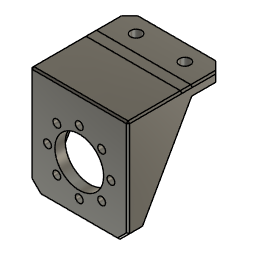
Simple Motor Bracket (Autodesk Fusion 360 design; units mm, degrees)
Autodesk Fusion 360 part; units mm, degrees
sketch "Sketch1" plane through (0, 0, 0) normal (0, 1, 0) x (1, 0, 0)
  circle A0 centre (0, 0) radius 7.5
  circle A1 centre (9.75, 0) radius 1.2
  line L0 (15, -14.8) -> (-15, -14.8)
  line L1 (-15, -14.8) -> (-15, 14.8)
  line L2 (-15, 14.8) -> (15, 14.8)
  line L3 (15, 14.8) -> (15, -14.8)
  line L4 (15, -14.8) -> (-15, 14.8) construction
  line L5 (-15, -14.8) -> (15, 14.8) construction
  line L6 (-15, -14.8) -> (-15, -18)
  line L7 (-15, -18) -> (15, -18)
  line L8 (15, -18) -> (15, -14.8)
  line L9 (12.8, 14.8) -> (12.8, -14.8)
  line L10 (0, 0) -> (0, -2.4)
  circle A2 centre (0, 0) radius 12.5
  circle A3 centre (0, 0) radius 9.75
  line L11 (0, 0) -> (9.75, 0)
  line L12 (1.75, 0) -> (22.5, 0)
  circle A4 centre (6.8943, -6.8943) radius 1.2
  line L13 (0, 0) -> (6.8943, -6.8943)
  line L14 (0, -1.75) -> (0, -22.5)
  circle A5 centre (-6.8943, -6.8943) radius 1.2
  circle A6 centre (-9.75, 0) radius 1.2
  circle A7 centre (0, -9.75) radius 1.2
  circle A8 centre (-6.8943, 6.8943) radius 1.2
  circle A9 centre (0, 9.75) radius 1.2
  circle A10 centre (6.8943, 6.8943) radius 1.2
  line L15 (-12.8, 14.8) -> (-12.8, -14.8)
  dimension "d1" = 15
  dimension "d3" = 2.4
  dimension "d6" = 30
  dimension "d7" = 29.6
  dimension "d8" = 3.2
  dimension "d30" = 2.2
  dimension "d38" = 25
  dimension "d39" = 19.5
  dimension "d40" = 45
  constraint coincident A0.centre L10.start
  constraint horizontal L0
  constraint perpendicular L0 L1
  constraint parallel L0 L2
  constraint parallel L1 L3
  constraint coincident L4 A0.centre
  constraint coincident L5 A0.centre
  constraint perpendicular L1 L7
  constraint perpendicular L6 L7
  constraint perpendicular L7 L8
  constraint coincident L2 L9.start
  constraint coincident L0 L9.end
  constraint perpendicular L0 L9
  constraint concentric A0 A3
  constraint coincident A1.centre A3
  constraint coincident A1.centre L11.end
  constraint parallel L11 L12
  constraint coincident A3 A4.centre
  constraint equal A1 A4
  constraint coincident A4.centre L13.end
  constraint symmetric A1 L14 A6
  constraint symmetric A4 L14 A5
  constraint coincident A3 A7.centre
  constraint coincident L14 A7.centre
  constraint equal A4 A7
  constraint symmetric L11 A4 A10
  constraint symmetric L11 A5 A8
  constraint symmetric L11 A7 A9
  constraint symmetric L9.start L10 L15.start
  constraint symmetric L9.end L10 L15.end
  constraint coincident L10.end L14
  measures "d1" diameter of A0
  measures "d3" diameter of A1
  measures "d6" distance of L1 L3
  measures "d7" distance of L0.start L2.end
  measures "d8" distance of L0 L7
  measures "d30" distance of L3 L9
  measures "d38" diameter of A2
  measures "d39" diameter of A3
  measures "d40" angle of L11 L13
extrude "Extrude1" add sketch "Sketch1" against normal blind 3.2 contours A0 A1 A3 L11 L12 A4 L13 | A0 A1 A3 L11 L12 L14 A5 A6 A7 A8 A9 A10 | A0 A3 A4 L13 L14 A7 | A1 A2 A3 L12 L14 A5 A6 A7 A8 A9 A10 | A1 A2 A3 L12 A4 L14 A7 | L0 L9 A2 L12 L14 | L0 L2 L9 A2 L12 L14 L15 | L0 L3 L9 L12 | L2 L3 L9 L12 | L0 L6 L7 L14 | L0 L7 L8 L14 | L0 L1 L2 L15
extrude "Extrude2" add sketch "Sketch1" along normal blind 26.8 contours L0 L6 L7 L14 | L0 L7 L8 L14
sketch "Sketch2" plane through (0, 0, 18) normal (0, 0, 1) x (-1, 0, 0)
  line L0 (15, -26.8) -> (15, 3.2)
  line L1 (15, 3.2) -> (-15, 3.2)
  line L2 (-15, 3.2) -> (-15, -26.8)
  line L3 (-15, -26.8) -> (15, -26.8)
  dimension "d29" = 0.5
sketch "Sketch3" plane through (0, 0, 18) normal (0, 0, 1) x (-1, 0, 0)
  circle A0 centre (7.5, -21.8) radius 1.7
  line L0 (15, 3.2) -> (-15, 3.2)
  line L1 (0, 0) -> (0, -4)
  circle A1 centre (-7.5, -21.8) radius 1.7
  line L2 (15, -13.4) -> (-15, -13.4)
  line L3 (-15, -13.4) -> (-15, -16.6)
  line L4 (-15, -16.6) -> (15, -16.6)
  line L5 (15, -16.6) -> (15, -13.4)
  line L6 (-15, -26.8) -> (15, -26.8)
  point P0 (-15, 3.2)
  dimension "d13" = 3.4
  dimension "d14" = 25
  dimension "d15" = 7.5
  dimension "d16" = 3.2
  dimension "d17" = 10.2
  constraint coincident L1.start origin
  constraint vertical L1
  constraint symmetric A0 L1 A1
  constraint horizontal L2
  constraint vertical L3
  constraint horizontal L4
  constraint vertical L5
  constraint collinear L0.start L2.start L4.end
  constraint collinear L2.end L3.end P0
  measures "d13" diameter of A0
  measures "d14" distance of A0.centre L0
  measures "d15" distance of A0.centre L1
  measures "d16" distance of L2 L4
  measures "d17" distance of L4 L6
extrude "Extrude3" cut sketch "Sketch3" against normal blind 3.2 contours A0 | A1
extrude "Extrude4" add sketch "Sketch3" along normal blind 0.01 contours L2 L3 L4 L5
extrude "Extrude6" add sketch "Sketch1" along normal blind 0.2 contours L0 L3 L9 L12 | L2 L3 L9 L12 | L0 L1 L2 L15
chamfer "Chamfer3" distance 16.5 distance2 29.5 3 edges at (13.9, 0.2, 14.8) (-13.9, 0.2, 14.8) (13.9, 0.2, 14.8) measured on face at (-2.2167, 6.9093, 14.8) measured on face at (-2.2167, 6.9093, 14.8) measured on face at (-2.2167, 6.9093, 14.8)
chamfer "Chamfer1" distance 3 angle 45 4 edges at (-15, 26.8, 16.4) (-15, -1.5, -14.8) (15, 26.8, 16.4) (15, -1.5, -14.8)
fillet "Fillet1" radius 0.5 1 edges at (0, 0, 14.8)
chamfer "Chamfer2" distance 0.5 angle 45 20 edges at (15, -3.2, 3.1) (15, 20.25, 14.8) (13.5, -3.2, -13.3) (0, -3.2, -14.8) (-13.5, -3.2, -13.3) (-15, -3.2, 3.1) (0, -3.2, 18) (-15, 20.25, 14.8) (-13.5, 25.3, 14.8) (0, 26.8, 14.8) (13.5, 25.3, 14.8) (0, 0, -14.8) (15, 9.261, 1.5) (-15, 9.261, 1.5) (15, 5.1, 18) (15, 15, 18.01) (15, 20.2, 18) (-15, 20.2, 18) (-15, 15, 18.01) (-15, 5.1, 18)
fillet "Fillet2" radius 0.5 3 edges at (12.8, 8.6, 14.8) (12.8, 0.1464, 14.6536) (12.8, 0, 0.15)
equation "d7 = 32.8 mm - 3.2 mm"
equation "d11 = 20 mm - 3.2 mm + 10 mm"
equation "d14 = 20 mm + 5 mm"
equation "d15 = ( 15 / 2 ) * 1 mm"
equation "d39 = ( ( 25 - 14 ) / 2 ) * 1 mm + 14 mm"
